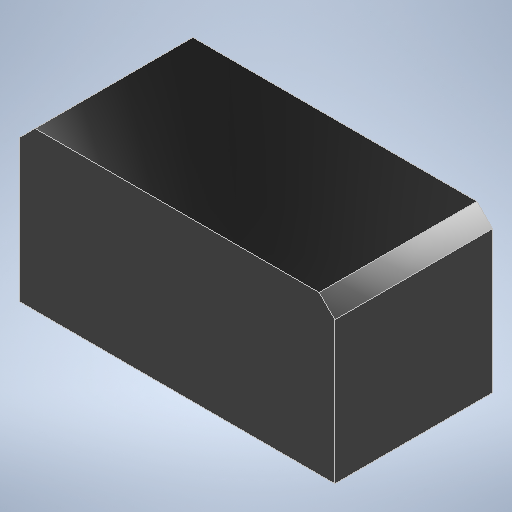
# Autodesk Inventor part: body
Saved by Autodesk Inventor 2025 (Build 290162000, 162)
## iProperties
Created: 2025-09-09
Part Number: body
Material: Phenolic Resin
Document SubType Name: Modeling
Designer: jirne
Density: 1.38 g/cm^3
Appearance: Smooth - Light Orange
Author: jirne
Autodesk Inventor part; units mm, degrees
ref_plane "YZ Plane" through (0, 0, 0) normal (1, 0, 0) x (0, 1, 0)
ref_plane "XZ Plane" through (0, 0, 0) normal (0, 1, 0) x (-1, 0, 0)
ref_plane "XY Plane" through (0, 0, 0) normal (0, 0, 1) x (1, 0, 0)
sketch "Sketch1" plane through (0, 0, 0) normal (0, 0, 1) x (1, 0, 0)
  line L0 (0, 0) -> (2.54, 0)
  line L1 (2.54, 0) -> (2.54, 1.27)
  line L2 (2.54, 1.27) -> (0, 1.27)
  line L3 (0, 1.27) -> (0, 0)
  dimension "d0" = 2.54
  dimension "d1" = 1.27
  constraints: 8 end point, 2 parallel, 1 horizontal, 1 perpendicular
  measures "d0" distance of L1.end L2.end
  measures "d1" distance of L0.end L1.end
extrude "Extrusion1" add sketch "Sketch1" along normal blind 1.27
chamfer "Chamfer1" distance 0.127 angle 45 2 edges at (0, 0.635, 1.27) (2.54, 0.635, 1.27)
body "Solid1"
